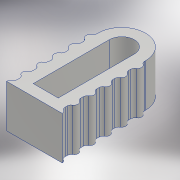
# Autodesk Inventor part: Tendeur
Saved by Autodesk Inventor 2017 (Build 210142000, 142)
## iProperties
Company: FABLAB Frenchmakers
Part Number: Tendeur
Material: Aluminium
Document SubType Name: Modeling
Designer: FABLAB Frenchmakers
Density: 2.7 g/cm^3
Appearance: Aluminium - Plat(2)
Mass: 0.741284 g
Surface Area: 4.77841 cm^2
Volume: 0.27455 cm^3
Project: 1420 Vauban 3D XL
Catalog Web Link: http://frenchmakers.com/
Stock Number: 1420-12-05
Autodesk Inventor part; units mm, degrees
ref_plane "YZ Plane" through (0, 0, 0) normal (1, 0, 0) x (0, 1, 0)
ref_plane "XZ Plane" through (0, 0, 0) normal (0, 1, 0) x (-1, 0, 0)
sketch "Esquisse1" plane through (0, 0, 0) normal (0, 0, 1) x (1, 0, 0)
  line L0 (-3, -7) -> (3, -7)
  line L1 (3, -7) -> (3, 4)
  line L2 (0, 7) -> (0, 7)
  line L3 (-3, 4) -> (-3, -7)
  line L4 (-3, -7) -> (3, 7) construction
  line L5 (3, -7) -> (-3, 7) construction
  arc A0 (0, 7) -> (-3, 4) centre (0, 4) ccw
  arc A1 (3, 4) -> (0, 7) centre (0, 4) ccw
  point P0 (0, 0)
  dimension "d0" = 6
  dimension "d1" = 14
  dimension "d2" = 3
  constraints: 12 end point, 4 point on circle, 4 point on line, 4 tangent, 2 centre point, 2 midpoint, 2 parallel, 1 concentric, 1 horizontal, 1 perpendicular
  measures "d0" distance of L5.end L4.end
  measures "d1" distance of L4.end L0.end
  measures "d2" radius of A0
extrude "Extrusion1" add sketch "Esquisse1" along normal mid plane 5.4
sketch "Esquisse2" plane through (0, 0, 2.7) normal (0, 0, 1) x (1, 0, 0)
  line L0 (-3, -7) -> (3, -7) construction
  line L1 (3, -7) -> (3, 4) construction
  arc A0 (3, 4) -> (-3, 4) centre (0, 4) ccw construction
  line L2 (-3, 4) -> (-3, -7) construction
  arc A1 (1.575, 4) -> (-1.575, 4) centre (0, 4) ccw
  line L3 (1.575, 4) -> (1.575, -5.575)
  line L4 (1.575, -5.575) -> (-1.575, -5.575)
  line L5 (-1.575, -5.575) -> (-1.575, 4)
  point P0 (0, 0)
  dimension "d21" = 3.15
  constraints: 6 end point, 2 point on circle, 1 centre point, 3 other
  measures "d21" distance between parallel lines of L3 L5
extrude "Extrusion2" cut sketch "Esquisse2" against normal through all
sketch "Esquisse3" plane through (0, 0, 2.7) normal (0, 0, 1) x (1, 0, 0)
  line L0 (3, 4) -> (3, -7) projected
  arc A0 (3.5, -7) -> (3, -6.5) centre (3, -7) ccw
  line L1 (-3, -7) -> (3, -7) projected
  line L2 (3, -7) -> (3.5, -7)
  line L3 (3, -7) -> (3, -6.5)
  arc A1 (3, -5.5) -> (3, -4.5) centre (3, -5) ccw
  arc A2 (3, -3.5) -> (3, -2.5) centre (3, -3) ccw
  arc A3 (3, -1.5) -> (3, -0.5) centre (3, -1) ccw
  arc A4 (3, 0.5) -> (3, 1.5) centre (3, 1) ccw
  arc A5 (3, 2.5) -> (3, 3.5) centre (3, 3) ccw
  line L4 (3, -5.5) -> (3, -4.5)
  line L5 (3, -3.5) -> (3, -2.5)
  line L6 (3, -1.5) -> (3, -0.5)
  line L7 (3, 0.5) -> (3, 1.5)
  line L8 (3, 2.5) -> (3, 3.5)
  point P0 (0, 0)
  dimension "d8" = 1
  dimension "d9" = 1
  dimension "d10" = 2
  dimension "d13" = 2
  constraints: 14 end point, 13 point on circle, 6 centre point, 6 point on line, 5 collinear, 1 horizontal, 1 vertical, 16 other
  measures "d8" diameter of A0
  measures "d9" diameter of A1
  measures "d10" distance of A0.centre A1.centre
  measures "d13" distance of A1.centre A2.centre
extrude "Extrusion3" add sketch "Esquisse3" against normal up to surface (5.4 mm away)
mirror "Symétrie1" about plane through (0, 0, 0) normal (1, 0, 0) of "Extrusion3"
fillet "Congé1" radius 0.5 33 edges at (3, -6.5, -1.35) (3, -6.5, 1.35) (3, -5.5, -1.35) (3, -4.5, -1.35) (3, -5.5, 1.35) (3, -4.5, 1.35) (3, -3.5, -1.35) (3, -2.5, -1.35) (3, -3.5, 1.35) (3, -2.5, 1.35) (3, -1.5, -1.35) (3, -0.5, -1.35) (3, -1.5, 1.35) (3, -0.5, 1.35) (3, 0.5, -1.35) (3, 1.5, -1.35) (3, 0.5, 1.35) (3, 1.5, 1.35) (3, 2.5, -1.35) (3, 3.5, -1.35) (3, 2.5, 1.35) (3, 3.5, 1.35) (-3, -6.5, 0) (-3, -4.5, 0) (-3, -5.5, 0) (-3, -2.5, 0) (-3, -3.5, 0) (-3, -0.5, 0) (-3, -1.5, 0) (-3, 1.5, 0) (-3, 0.5, 0) (-3, 3.5, 0) (-3, 2.5, 0)
ref_plane "Plan de construction1" through (3.5, 4, -2.7) normal (0, -1, 0) x (1, 0, 0)
equation "\"d9\" = d8"
